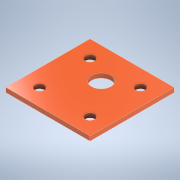
# Autodesk Inventor part: pcb
Saved by Autodesk Inventor 2022 (Build 260153000, 153)
## iProperties
Created: 2022-04-20
Part Number: pcb
Material: フェノール樹脂
Document SubType Name: Modeling
Designer: Yazawa
Density: 1.38 g/cm^3
Appearance: 滑らか - 淡いオレンジ
Author: Yazawa
Autodesk Inventor part; units mm, degrees
ref_plane "YZ Plane" through (0, 0, 0) normal (1, 0, 0) x (0, 1, 0)
ref_plane "XZ Plane" through (0, 0, 0) normal (0, 1, 0) x (-1, 0, 0)
ref_plane "XY Plane" through (0, 0, 0) normal (0, 0, 1) x (1, 0, 0)
sketch "スケッチ1" plane through (0, 0, 0) normal (0, 1, 0) x (-1, 0, 0)
  line L0 (15, -15) -> (-15, -15)
  line L1 (-15, -15) -> (-15, 15)
  line L2 (-15, 15) -> (15, 15)
  line L3 (15, 15) -> (15, -15)
  line L4 (15, -15) -> (-15, 15) construction
  line L5 (-15, -15) -> (15, 15) construction
  point P0 (0, 0)
  point P1 (0, 0)
  dimension "d0" = 30
  dimension "d1" = 30
  constraints: 12 end point, 2 parallel, 1 coincident, 1 horizontal, 1 midpoint, 1 perpendicular
  measures "d0" distance of L1.end L2.end
  measures "d1" distance of L0.end L1.end
extrude "押し出し1" add sketch "スケッチ1" along normal blind 1.6
sketch "スケッチ3" plane through (0, 1.6, 0) normal (0, 1, 0) x (1, 0, 0)
  point P0 (0, 0)
  point P1 (0, 4)
  dimension "d17" = 4
  measures "d17" distance of point (0, 4) point (0, 0)
hole "穴2" at (0, 1.6, -4) direction (0, -1, 0) diameter 7 depth 4.8
sketch "スケッチ4" plane through (0, 1.6, 0) normal (0, 1, 0) x (1, 0, 0)
  line L0 (15, 15) -> (-15, 15) projected
  line L1 (15, -15) -> (15, 15) projected
  point P0 (0, 0)
  point P1 (-9, -9)
  point P2 (9, -9)
  point P3 (9, 9)
  point P4 (-9, 9)
  dimension "d27" = 360
  dimension "d36" = 6
  dimension "d37" = 6
  constraints: 5 other
  measures "d36" distance from line of L0 point (9, 9)
  measures "d37" distance from line of L1 point (9, 9)
hole "穴3" at (-9, 1.6, 9) at (9, 1.6, 9) at (9, 1.6, -9) at (-9, 1.6, -9) direction (0, -1, 0) diameter 3.4036 depth 1.6 clearance for "Countersunk Flat Head Screw ISO 2009/7046" size "M3" standard "ISO"
